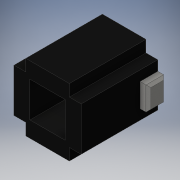
# Autodesk Inventor part: MotorBody
Saved by Autodesk Inventor 2016 (Build 200138000, 138)
## iProperties
Created: 2016-11-29
Part Number: MotorBody
Material: Generic
Document SubType Name: Modeling
Designer: Evan Phil George
Density: 1 g/cm^3
Appearance: Default
Author: Evan Phil George
Autodesk Inventor part; units mm, degrees
ref_plane "YZ Plane" through (0, 0, 0) normal (1, 0, 0) x (0, 1, 0)
ref_plane "XZ Plane" through (0, 0, 0) normal (0, 1, 0) x (-1, 0, 0)
ref_plane "XY Plane" through (0, 0, 0) normal (0, 0, 1) x (1, 0, 0)
sketch "Sketch1" plane through (0, 0, 0) normal (0, 0, 1) x (1, 0, 0)
  line L0 (-28.5, 28.5) -> (28.5, 28.5)
  line L1 (28.5, 28.5) -> (28.5, -28.5)
  line L2 (28.5, -28.5) -> (-28.5, -28.5)
  line L3 (-28.5, -28.5) -> (-28.5, 28.5)
  line L4 (-15, 15) -> (15, 15)
  line L5 (15, 15) -> (15, -15)
  line L6 (15, -15) -> (-15, -15)
  line L7 (-15, -15) -> (-15, 15)
  line L8 (-18.5, 28.5) -> (-18.5, 18.5)
  line L9 (-18.5, 18.5) -> (-28.5, 18.5)
  line L10 (18.5, 28.5) -> (18.5, 18.5)
  line L11 (18.5, 18.5) -> (28.5, 18.5)
  line L12 (28.5, -18.5) -> (18.5, -18.5)
  line L13 (18.5, -18.5) -> (18.5, -28.5)
  line L14 (-28.5, -18.5) -> (-18.5, -18.5)
  line L15 (-18.5, -18.5) -> (-18.5, -28.5)
  line L16 (-18.5, 28.5) -> (18.5, 28.5)
  line L17 (28.5, 18.5) -> (28.5, -18.5)
  line L18 (18.5, -28.5) -> (-18.5, -28.5)
  line L19 (-28.5, -18.5) -> (-28.5, 18.5)
  point P0 (0, 0)
  dimension "d0" = 28.5
  dimension "d1" = 28.5
  dimension "d2" = 57
  dimension "d3" = 57
  dimension "d4" = 30
  dimension "d5" = 30
  dimension "d6" = 15
  dimension "d7" = 15
  dimension "d8" = 10
  dimension "d9" = 10
  dimension "d10" = 10
  dimension "d11" = 10
  dimension "d12" = 10
  dimension "d13" = 10
  dimension "d14" = 10
  constraints: 40 end point, 10 point on line, 6 perpendicular, 4 parallel, 3 collinear, 3 horizontal, 3 vertical
  measures "d0" distance from line of point (0, 0) L0
  measures "d1" distance from line of point (0, 0) L1
  measures "d2" distance of L0.start L0.end
  measures "d3" distance of L0.end L1.end
  measures "d4" distance of L4.start L4.end
  measures "d5" distance of L4.end L5.end
  measures "d6" distance from line of point (0, 0) L4
  measures "d7" distance from line of point (0, 0) L5
  measures "d8" distance of L8.start L8.end
  measures "d9" distance of L8.end L9.end
  measures "d10" distance of L10.start L10.end
  measures "d11" distance of L10.end L11.end
  measures "d12" distance of L12.start L12.end
  measures "d13" distance of L12.end L13.end
  measures "d14" distance of L14.start L14.end
extrude "Extrusion1" add sketch "Sketch1" along normal mid plane 65 contours L0 L10 L11 L1 L12 L13 L2 L15 L14 L3 L9 L8
sketch "Sketch2" plane through (28.5, -18.5, 32.5) normal (1, 0, 0) x (0, 0, -1)
  line L0 (65, 33.5) -> (65, 3.5) projected
  line L1 (65, 18.5) -> (65, 28.5)
  line L2 (65, 28.5) -> (50, 28.5)
  line L3 (50, 28.5) -> (50, 8.5)
  line L4 (50, 8.5) -> (65, 8.5)
  point P0 (32.5, 18.5)
  dimension "d17" = 10
  dimension "d20" = 15
  dimension "d22" = 20
  constraints: 8 end point, 2 perpendicular, 2 point on line, 1 midpoint, 1 vertical
  measures "d17" distance of L1.start L1.end
  measures "d20" distance of L1.end L2.end
  measures "d22" distance of L2.end L3.end
extrude "Extrusion2" add sketch "Sketch2" along normal blind 7
chamfer "Chamfer1" distance 2 angle 45 4 edges at (35.5, 10, -25) (35.5, 0, -32.5) (35.5, -10, -25) (35.5, 0, -17.5)
body "Solid1"
